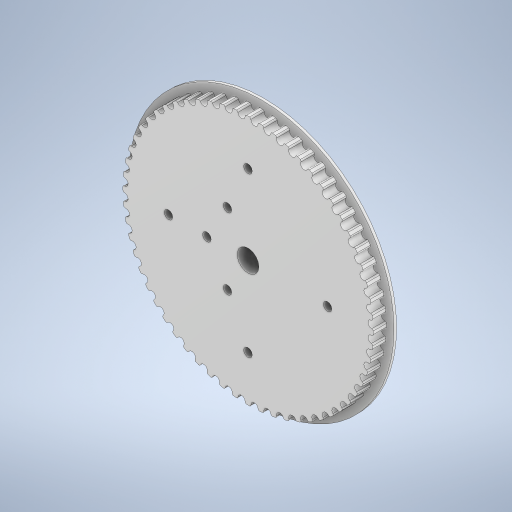
# Autodesk Inventor part: 射出_プーリ_歯数60
Saved by Autodesk Inventor 2023 (Build 270158000, 158)
## iProperties
Created: 2022-02-01
Part Number: 射出_プーリ_歯数60
Material: アセタール樹脂、白
Document SubType Name: Modeling
Designer: hirohumi
Density: 1.425 g/cm^3
Appearance: 滑らか - 白
Author: hirohumi
Autodesk Inventor part; units mm, degrees
ref_plane "YZ Plane" through (0, 0, 0) normal (1, 0, 0) x (0, 1, 0)
ref_plane "XZ Plane" through (0, 0, 0) normal (0, 1, 0) x (-1, 0, 0)
ref_plane "XY Plane" through (0, 0, 0) normal (0, 0, 1) x (1, 0, 0)
sketch "スケッチ1" plane through (0, 0, 0) normal (0, 0, 1) x (1, 0, 0)
  arc A0 (11.2031, 43.8361) -> (-12.7392, 43.4146) centre (0, 0) ccw construction
  arc A1 (-0.569, 47.1716) -> (-1.072, 46.6316) centre (-0.5629, 46.6616) ccw
  arc A2 (1.072, 46.6316) -> (0.569, 47.1716) centre (0.5629, 46.6616) ccw
  arc A3 (-2.3679, 45.183) -> (-1.072, 46.6316) centre (-2.4396, 46.5511) ccw
  arc A4 (1.072, 46.6316) -> (2.3679, 45.183) centre (2.4396, 46.5511) ccw
  arc A5 (0.569, 47.1716) -> (-0.569, 47.1716) centre (0, 0) ccw
  line L0 (-2.3679, 45.183) -> (0, 0)
  line L1 (0, 0) -> (2.3679, 45.183)
  line L2 (0, 0) -> (0, 8.5337) construction
  dimension "d4" = 0.51
  dimension "d5" = 0.51
  dimension "d6" = 1.37
  dimension "d7" = 1.37
  dimension "d8" = 6
  dimension "d9" = 3
  dimension "d20" = 47.175
  dimension "d21" = 1.93
  constraints: 14 point on circle, 6 centre point, 6 end point, 6 tangent, 2 coincident, 1 vertical
  measures "d4" radius of A1
  measures "d5" radius of A2
  measures "d6" radius of A3
  measures "d7" radius of A4
  measures "d8" angle of L1 L0
  measures "d9" angle of L2 L0
  measures "d20" radius of A5
  measures "d21" radial gap between concentric circles of A0 A5
extrude "押し出し1" add sketch "スケッチ1" along normal blind 5
pattern_circular "円形状パターン1" count 60 over 360 about axis through (0, 0, 0) along (0, 0, 1) of "押し出し1"
sketch "スケッチ2" plane through (0, 0, 0) normal (0, 0, -1) x (-1, 0, 0)
  circle A0 centre (0, 0) radius 50
  dimension "d15" = 100
  constraints: 1 centre point, 1 coincident
  measures "d15" diameter of A0
extrude "押し出し2" add sketch "スケッチ2" along normal blind 1
sketch "スケッチ5" plane through (0, 0, 5) normal (0, 0, 1) x (1, 0, 0)
  circle A0 centre (0, 0) radius 6.1 projected
  circle A1 centre (0, 0) radius 30 construction
  point P0 (-30, 0)
  point P1 (0, 30)
  point P2 (30, 0)
  point P3 (0, -30)
  dimension "d40" = 60
  constraints: 4 point on circle, 1 centre point, 1 coincident
  measures "d40" diameter of A1
hole "穴1" at (-30, 0, 5) at (0, 30, 5) at (30, 0, 5) at (0, -30, 5) direction (0, 0, -1) diameter 3.2 end through all
sketch "スケッチ7" plane through (0, 0, 5) normal (0, 0, 1) x (1, 0, 0)
  circle A0 centre (0, 0) radius 4.1
  circle A1 centre (-15.5, 0) radius 1.6
  line L0 (0, 0) -> (-13.1555, 22.7859) construction
  line L1 (0, 0) -> (26.3109, 0) construction
  circle A2 centre (0, 0) radius 15.5 construction
  line L2 (0, 0) -> (-9.6332, -16.6852) construction
  line L3 (0, 0) -> (19.2664, 0) construction
  circle A3 centre (-7.75, 13.4234) radius 1.6
  circle A4 centre (-7.75, -13.4234) radius 1.6
  dimension "d60" = 8.2
  dimension "d61" = 3.2
  dimension "d62" = 15.5
  dimension "d64" = 120
  dimension "d65" = 31
  dimension "d66" = 120
  dimension "d67" = 3.2
  dimension "d68" = 3.2
  constraints: 8 end point, 5 centre point, 2 coincident, 2 equal length, 2 horizontal, 2 point on circle, 2 point on line
  measures "d60" diameter of A0
  measures "d61" diameter of A1
  measures "d62" distance of A1.centre point (0, 0)
  measures "d64" angle of L1 L0
  measures "d65" diameter of A2
  measures "d66" angle of L2 L3
  measures "d67" diameter of A3
  measures "d68" diameter of A4
extrude "押し出し6" cut sketch "スケッチ7" against normal blind 10
